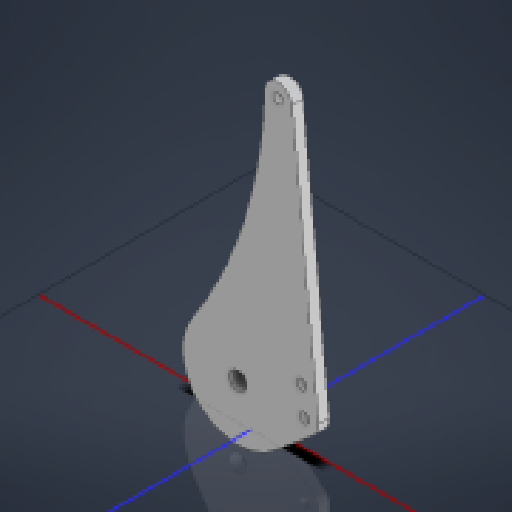
# Autodesk Inventor part: intakeSide
Saved by Autodesk Inventor 2025.2 (Build 292293000, 293)
## iProperties
Created: 2025-12-05
Part Number: intakeSide
Material: Generic
Document SubType Name: Modeling
Designer: cloudy
Density: 1 g/cm^3
Appearance: Default
Author: cloudy
Autodesk Inventor part; units mm, degrees
ref_plane "YZ Plane" through (0, 0, 0) normal (1, 0, 0) x (0, 1, 0)
ref_plane "XZ Plane" through (0, 0, 0) normal (0, 1, 0) x (-1, 0, 0)
ref_plane "XY Plane" through (0, 0, 0) normal (0, 0, 1) x (1, 0, 0)
sketch "Sketch1" plane through (0, 0, 0) normal (0, 0, 1) x (1, 0, 0)
  circle A0 centre (1.835, -47.1215) radius 2.1844
  circle A1 centre (12.7, 69.85) radius 2.1844 projected
  arc A2 (19.0097, 70.5645) -> (6.3511, 69.7333) centre (12.7, 69.85) ccw
  arc A3 (-20.2372, -34.5525) -> (25.9922, -54.9693) centre (1.835, -47.1215) ccw
  line L0 (25.9922, -54.9693) -> (30.9301, -39.7696)
  line L1 (31.2005, -37.0931) -> (19.0097, 70.5645)
  arc A4 (-20.2372, -34.5525) -> (6.3511, 69.7333) centre (-196.8146, 65.9992) ccw
  arc A5 (30.9301, -39.7696) -> (31.2005, -37.0931) centre (24.8908, -37.8076) ccw
  line L2 (5.0608, -43.8957) -> (-1.3908, -43.8957)
  line L3 (-1.3908, -43.8957) -> (-1.3908, -50.3473)
  line L4 (-1.3908, -50.3473) -> (5.0608, -50.3473)
  line L5 (5.0608, -50.3473) -> (5.0608, -43.8957)
  line L6 (5.0608, -43.8957) -> (-1.3908, -50.3473) construction
  line L7 (-1.3908, -43.8957) -> (5.0608, -50.3473) construction
  circle A6 centre (1.835, -47.1215) radius 3.937
  circle A7 centre (24.8908, -37.8076) radius 2.1844
  circle A8 centre (23.4618, -25.1883) radius 2.1844
  line L8 (24.8908, -37.8076) -> (23.4618, -25.1883)
  line L9 (1.835, -47.1215) -> (12.7, 69.85)
  point P0 (0, 0)
  dimension "d0" = 12.7
  dimension "d2" = 50.8
  dimension "d3" = 203.2
  dimension "d4" = 6.35
  dimension "d7" = 6.4516
  dimension "d8" = 6.4516
  dimension "d10" = 7.874
  dimension "d11" = 4.3688
  dimension "d12" = 4.3688
  dimension "d14" = 12.7
  dimension "d15" = 117.475
  constraints: 20 end point, 8 centre point, 8 point on circle, 6 tangent, 4 coincident, 3 parallel, 2 midpoint, 1 horizontal, 1 perpendicular
  measures "d0" diameter of A2
  measures "d2" diameter of A3
  measures "d3" radius of A4
  measures "d4" radius of A5
  measures "d7" distance of L4.end L3.end
  measures "d8" distance of L3.end L2.end
  measures "d10" diameter of A6
  measures "d11" diameter of A7
  measures "d12" diameter of A8
  measures "d14" distance of L8.start L8.end
  measures "d15" distance of L9.start L9.end
extrude "Extrusion1" add sketch "Sketch1" along normal blind 5.08 contours L2 L5 A6 | A6 L3 L2 | L5 L4 A6 | A6 L4 L3 | L1 A5 L0 A3 A4 A2
body "Solid1"
